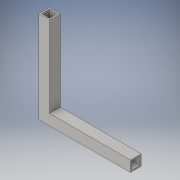
# Autodesk Inventor part: 60DegreeAlumTubing
Saved by Autodesk Inventor 2016 SP1 (Build 200210100, 210)
## iProperties
Created: 2016-01-25
Part Number: 60DegreeAlumTubing
Material: Generic
Document SubType Name: Modeling
Designer: steele
Density: 1 g/cm^3
Appearance: Default
Author: steele
Autodesk Inventor part; units mm, degrees
ref_plane "YZ Plane" through (0, 0, 0) normal (1, 0, 0) x (0, 1, 0)
ref_plane "XZ Plane" through (0, 0, 0) normal (0, 1, 0) x (-1, 0, 0)
ref_plane "XY Plane" through (0, 0, 0) normal (0, 0, 1) x (1, 0, 0)
sketch "Sketch1" plane through (0, 0, 0) normal (0, 0, 1) x (1, 0, 0)
  line L0 (0, 0) -> (-203.2, 0)
  line L1 (-203.2, 0) -> (-203.2, 203.2)
  dimension "d0" = 90
  dimension "d1" = 203.2
  constraints: 4 end point, 1 horizontal, 1 perpendicular
  measures "d0" angle of L1 L0
  measures "d1" distance of L0.start L0.end
sketch "Sketch2" plane through (0, 0, 0) normal (1, 0, 0) x (0, 1, 0)
  line L0 (-12.7, 12.7) -> (-12.7, -12.7)
  line L1 (-12.7, -12.7) -> (12.7, -12.7)
  line L2 (12.7, -12.7) -> (12.7, 12.7)
  line L3 (12.7, 12.7) -> (-12.7, 12.7)
  line L4 (-12.7, 12.7) -> (12.7, -12.7) construction
  line L5 (-12.7, -12.7) -> (12.7, 12.7) construction
  line L6 (-9.525, 9.525) -> (-9.525, -9.525)
  line L7 (-9.525, -9.525) -> (9.525, -9.525)
  line L8 (9.525, -9.525) -> (9.525, 9.525)
  line L9 (9.525, 9.525) -> (-9.525, 9.525)
  line L10 (-9.525, 9.525) -> (9.525, -9.525) construction
  line L11 (-9.525, -9.525) -> (9.525, 9.525) construction
  point P0 (0, 0)
  dimension "d2" = 25.4
  dimension "d3" = 3.175
  constraints: 24 end point, 4 midpoint, 4 parallel, 4 perpendicular, 2 vertical
  measures "d2" distance of L0.start L0.end
  measures "d3" distance between parallel lines of L0 L6
sweep "Sweep1" add profiles "Sketch2" path "Sketch1"
body "Solid1"
